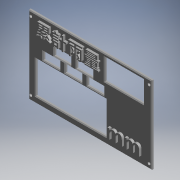
# Autodesk Inventor part: 雨量
Saved by Autodesk Inventor 2021 (Build 250183000, 183)
## iProperties
Part Number: 雨量
Material: 一般
Document SubType Name: 塑型
Designer: aura0
Appearance: 預設
Author: aura0
Autodesk Inventor part; units mm, degrees
ref_plane "YZ 平面" through (0, 0, 0) normal (1, 0, 0) x (0, 1, 0)
ref_plane "XZ 平面" through (0, 0, 0) normal (0, 1, 0) x (-1, 0, 0)
ref_plane "XY 平面" through (0, 0, 0) normal (0, 0, 1) x (1, 0, 0)
sketch "草圖1" plane through (0, 0, 0) normal (0, 0, 1) x (1, 0, 0)
  line L0 (-81, -51) -> (81, -51)
  line L1 (81, -51) -> (81, 51)
  line L2 (81, 51) -> (-81, 51)
  line L3 (-81, 51) -> (-81, -51)
  line L4 (-81, -51) -> (81, 51) construction
  line L5 (81, -51) -> (-81, 51) construction
  point P0 (0, 0)
  dimension "d0" = 162
  dimension "d1" = 102
  constraints: 12 end point, 2 midpoint, 2 parallel, 1 horizontal, 1 perpendicular
  measures "d0" distance of L2.end L1.end
  measures "d1" distance of L1.end L0.end
extrude "擠出1" add sketch "草圖1" along normal blind 3
sketch "草圖2" plane through (0, 0, 3) normal (0, 0, 1) x (1, 0, 0)
  line L0 (-72, -43) -> (21, -43)
  line L1 (21, -43) -> (21, 0)
  line L2 (21, 0) -> (-72, 0)
  line L3 (-72, 0) -> (-72, -43)
  line L4 (-62, 2.8) -> (-40, 2.8)
  line L5 (-40, 2.8) -> (-40, 13)
  line L6 (-40, 13) -> (-62, 13)
  line L7 (-62, 13) -> (-62, 2.8)
  line L8 (-33, 2.8) -> (-11, 2.8)
  line L9 (-11, 2.8) -> (-11, 13)
  line L10 (-11, 13) -> (-33, 13)
  line L11 (-33, 13) -> (-33, 2.8)
  line L12 (-4, 2.8) -> (18, 2.8)
  line L13 (18, 2.8) -> (18, 13)
  line L14 (18, 13) -> (-4, 13)
  line L15 (-4, 13) -> (-4, 2.8)
  line L16 (-47.5, 15) -> (-25.5, 15)
  line L17 (-25.5, 15) -> (-25.5, 25.2)
  line L18 (-25.5, 25.2) -> (-47.5, 25.2)
  line L19 (-47.5, 25.2) -> (-47.5, 15)
  line L20 (-18.5, 15) -> (3.5, 15)
  line L21 (3.5, 15) -> (3.5, 25.2)
  line L22 (3.5, 25.2) -> (-18.5, 25.2)
  line L23 (-18.5, 25.2) -> (-18.5, 15)
  line L24 (19, 19) -> (70, 19)
  line L25 (70, 19) -> (70, 47)
  line L26 (70, 47) -> (19, 47)
  line L27 (19, 47) -> (19, 19)
  line L28 (-81, -51) -> (81, -51) projected
  line L29 (-81, 51) -> (-81, -51) projected
  point P0 (0, 0)
  dimension "d4" = 8
  dimension "d5" = 9
  dimension "d6" = 43
  dimension "d7" = 93
  dimension "d8" = 53.8
  dimension "d9" = 19
  dimension "d10" = 22
  dimension "d11" = 10.2
  dimension "d12" = 0
  dimension "d13" = 0
  dimension "d14" = 22
  dimension "d15" = 7
  dimension "d16" = 7
  dimension "d17" = 22
  dimension "d18" = 10.2
  dimension "d19" = 10.2
  dimension "d20" = 66
  dimension "d21" = 33.5
  dimension "d22" = 22
  dimension "d23" = 10.2
  dimension "d24" = 0
  dimension "d25" = 7
  dimension "d26" = 22
  dimension "d27" = 10.2
  dimension "d28" = 70
  dimension "d29" = 100
  dimension "d30" = 51
  dimension "d31" = 28
  constraints: 56 end point, 14 parallel, 7 horizontal, 7 perpendicular
  measures "d4" distance between parallel lines of L28 L0
  measures "d5" distance between parallel lines of L29 L3
  measures "d6" distance of L0.end L1.end
  measures "d7" distance of L0.start L0.end
  measures "d8" distance between parallel lines of L28 L4
  measures "d9" distance between parallel lines of L29 L7
  measures "d10" distance of L4.start L4.end
  measures "d11" distance of L4.end L5.end
  measures "d12" distance between parallel lines of L4 L8
  measures "d13" distance between parallel lines of L4 L12
  measures "d14" distance of L8.start L8.end
  measures "d15" distance between parallel lines of L5 L11
  measures "d16" distance between parallel lines of L15 L9
  measures "d17" distance of L12.start L12.end
  measures "d18" distance of L8.end L9.end
  measures "d19" distance of L12.end L13.end
  measures "d20" distance between parallel lines of L28 L16
  measures "d21" distance between parallel lines of L29 L19
  measures "d22" distance of L16.start L16.end
  measures "d23" distance of L16.end L17.end
  measures "d24" distance between parallel lines of L16 L20
  measures "d25" distance between parallel lines of L23 L17
  measures "d26" distance of L20.start L20.end
  measures "d27" distance of L20.end L21.end
  measures "d28" distance between parallel lines of L28 L24
  measures "d29" distance between parallel lines of L27 L29
  measures "d30" distance of L24.start L24.end
  measures "d31" distance of L24.end L25.end
extrude "擠出2" cut sketch "草圖2" against normal blind 3
sketch "草圖3" plane through (0, 0, 3) normal (0, 0, 1) x (1, 0, 0)
  line L0 (-69.5952, 46.7883) -> (36.1559, 46.7883) construction
  line L1 (36.1559, 46.7883) -> (36.1559, 23.2347) construction
  line L2 (36.1559, 23.2347) -> (-69.5952, 23.2347) construction
  line L3 (-69.5952, 23.2347) -> (-69.5952, 46.7883) construction
  line L4 (23.9815, -27.7989) -> (32.0649, -27.7989) construction
  line L5 (32.0649, -27.7989) -> (32.0649, -30.4991) construction
  line L6 (32.0649, -30.4991) -> (23.9815, -30.4991) construction
  line L7 (23.9815, -30.4991) -> (23.9815, -27.7989) construction
  line L8 (-50.1617, 32.9995) -> (-51.6312, 31.9832)
  spline S0 degree 2 poles (-51.6312, 31.9832) (-52.2355, 32.7935) (-52.7574, 33.3016) knots 0 0 0 1 1 1
  spline S1 degree 2 poles (-52.7574, 33.3016) (-55.1609, 33.0132) (-57.9214, 32.8759) knots 0 0 0 1 1 1
  line L9 (-57.9214, 32.8759) -> (-57.9214, 30.0467)
  spline S2 degree 2 poles (-57.9214, 30.0467) (-57.9214, 29.2776) (-58.8553, 28.1377) (-60.6682, 28.1377) knots 0 0 0 1 2 2 2
  spline S3 degree 2 poles (-60.6682, 28.1377) (-61.1626, 28.1377) (-61.6158, 28.1789) knots 0 0 0 1 1 1
  line L10 (-61.6158, 28.1789) -> (-62.2338, 29.7858)
  spline S4 degree 2 poles (-62.2338, 29.7858) (-60.8467, 29.7583) (-59.7892, 29.8407) (-59.7892, 30.2939) knots 0 0 0 1 2 2 2
  line L11 (-59.7892, 30.2939) -> (-59.7892, 32.7248)
  spline S5 degree 2 poles (-59.7892, 32.7248) (-63.4012, 32.4913) (-66.7797, 32.4913) knots 0 0 0 1 1 1
  line L12 (-66.7797, 32.4913) -> (-67.1231, 34.0021)
  spline S6 degree 2 poles (-67.1231, 34.0021) (-64.1566, 34.263) (-59.8716, 36.0759) knots 0 0 0 1 1 1
  spline S7 degree 2 poles (-59.8716, 36.0759) (-64.5411, 35.6639) (-65.5574, 35.6227) knots 0 0 0 1 1 1
  line L13 (-65.5574, 35.6227) -> (-65.7909, 37.1059)
  spline S8 degree 2 poles (-65.7909, 37.1059) (-63.6484, 37.5729) (-61.5197, 39.0424) knots 0 0 0 1 1 1
  line L14 (-61.5197, 39.0424) -> (-66.3815, 39.0424)
  line L15 (-66.3815, 39.0424) -> (-66.3815, 46.239)
  line L16 (-66.3815, 46.239) -> (-51.4527, 46.239)
  line L17 (-51.4527, 46.239) -> (-51.4527, 39.0424)
  line L18 (-51.4527, 39.0424) -> (-58.8965, 39.0424)
  spline S9 degree 2 poles (-58.8965, 39.0424) (-60.3385, 37.9025) (-61.8081, 37.2158) knots 0 0 0 1 1 1
  spline S10 degree 2 poles (-61.8081, 37.2158) (-60.833, 37.2433) (-58.9102, 37.3806) (-56.4793, 37.6415) (-55.5729, 38.1222) (-54.8724, 38.548) knots 0 0 0 1 2 3 4 4 4
  line L19 (-54.8724, 38.548) -> (-53.2656, 37.669)
  spline S11 degree 2 poles (-53.2656, 37.669) (-57.5368, 35.3343) (-62.0003, 34.0021) knots 0 0 0 1 1 1
  spline S12 degree 2 poles (-62.0003, 34.0021) (-58.0587, 34.1257) (-54.1308, 34.6064) knots 0 0 0 1 1 1
  spline S13 degree 2 poles (-54.1308, 34.6064) (-54.2956, 34.7986) (-55.0235, 35.4167) knots 0 0 0 1 1 1
  line L20 (-55.0235, 35.4167) -> (-53.5265, 36.378)
  spline S14 degree 2 poles (-53.5265, 36.378) (-51.5488, 34.7574) (-50.1617, 32.9995) knots 0 0 0 1 1 1
  line L21 (-49.5849, 29.7583) -> (-50.7111, 28.3712)
  spline S15 degree 2 poles (-50.7111, 28.3712) (-53.293, 29.9231) (-56.6167, 31.0493) knots 0 0 0 1 1 1
  line L22 (-56.6167, 31.0493) -> (-55.2982, 32.3815)
  spline S16 degree 2 poles (-55.2982, 32.3815) (-51.9883, 31.2553) (-49.5849, 29.7583) knots 0 0 0 1 1 1
  spline S17 degree 2 poles (-61.0939, 31.2003) (-63.4699, 29.6347) (-67.1643, 28.4536) knots 0 0 0 1 1 1
  line L23 (-67.1643, 28.4536) -> (-68.2767, 29.978)
  spline S18 degree 2 poles (-68.2767, 29.978) (-64.9531, 30.8845) (-62.7145, 32.2441) knots 0 0 0 1 1 1
  line L24 (-62.7145, 32.2441) -> (-61.0939, 31.2003)
  line L25 (-53.3342, 43.3823) -> (-53.3342, 44.6596)
  line L26 (-53.3342, 44.6596) -> (-58.0038, 44.6596)
  line L27 (-58.0038, 44.6596) -> (-58.0038, 43.3823)
  line L28 (-58.0038, 43.3823) -> (-53.3342, 43.3823)
  line L29 (-53.3342, 40.663) -> (-53.3342, 41.9265)
  line L30 (-53.3342, 41.9265) -> (-58.0038, 41.9265)
  line L31 (-58.0038, 41.9265) -> (-58.0038, 40.663)
  line L32 (-58.0038, 40.663) -> (-53.3342, 40.663)
  line L33 (-59.8853, 43.3823) -> (-59.8853, 44.6596)
  line L34 (-59.8853, 44.6596) -> (-64.4587, 44.6596)
  line L35 (-64.4587, 44.6596) -> (-64.4587, 43.3823)
  line L36 (-64.4587, 43.3823) -> (-59.8853, 43.3823)
  line L37 (-59.8853, 40.663) -> (-59.8853, 41.9265)
  line L38 (-59.8853, 41.9265) -> (-64.4587, 41.9265)
  line L39 (-64.4587, 41.9265) -> (-64.4587, 40.663)
  line L40 (-64.4587, 40.663) -> (-59.8853, 40.663)
  line L41 (-28.5583, 38.9463) -> (-32.4175, 38.9463)
  line L42 (-32.4175, 38.9463) -> (-32.4175, 28.1789)
  line L43 (-32.4175, 28.1789) -> (-34.3403, 28.1789)
  line L44 (-34.3403, 28.1789) -> (-34.3403, 38.9463)
  line L45 (-34.3403, 38.9463) -> (-38.1033, 38.9463)
  line L46 (-38.1033, 38.9463) -> (-38.1033, 40.8003)
  line L47 (-38.1033, 40.8003) -> (-34.3403, 40.8003)
  line L48 (-34.3403, 40.8003) -> (-34.3403, 46.6235)
  line L49 (-34.3403, 46.6235) -> (-32.4175, 46.6235)
  line L50 (-32.4175, 46.6235) -> (-32.4175, 40.8003)
  line L51 (-32.4175, 40.8003) -> (-28.5583, 40.8003)
  line L52 (-28.5583, 40.8003) -> (-28.5583, 38.9463)
  line L53 (-39.1746, 28.4536) -> (-41.0149, 28.4536)
  line L54 (-41.0149, 28.4536) -> (-41.0149, 29.5111)
  line L55 (-41.0149, 29.5111) -> (-44.2973, 29.5111)
  line L56 (-44.2973, 29.5111) -> (-44.2973, 28.1789)
  line L57 (-44.2973, 28.1789) -> (-46.1651, 28.1789)
  line L58 (-46.1651, 28.1789) -> (-46.1651, 35.4579)
  line L59 (-46.1651, 35.4579) -> (-39.1746, 35.4579)
  line L60 (-39.1746, 35.4579) -> (-39.1746, 28.4536)
  line L61 (-38.227, 43.039) -> (-47.0304, 43.039)
  line L62 (-47.0304, 43.039) -> (-47.0304, 44.7145)
  line L63 (-47.0304, 44.7145) -> (-43.542, 44.7145)
  spline S19 degree 2 poles (-43.542, 44.7145) (-43.8853, 45.6072) (-44.3248, 46.4312) knots 0 0 0 1 1 1
  line L64 (-44.3248, 46.4312) -> (-42.3471, 46.7883)
  spline S20 degree 2 poles (-42.3471, 46.7883) (-41.8664, 45.9368) (-41.427, 44.7145) knots 0 0 0 1 1 1
  line L65 (-41.427, 44.7145) -> (-38.227, 44.7145)
  line L66 (-38.227, 44.7145) -> (-38.227, 43.039)
  line L67 (-39.2158, 39.8939) -> (-46.2613, 39.8939)
  line L68 (-46.2613, 39.8939) -> (-46.2613, 41.5832)
  line L69 (-46.2613, 41.5832) -> (-39.2158, 41.5832)
  line L70 (-39.2158, 41.5832) -> (-39.2158, 39.8939)
  line L71 (-39.2158, 36.845) -> (-46.2613, 36.845)
  line L72 (-46.2613, 36.845) -> (-46.2613, 38.5205)
  line L73 (-46.2613, 38.5205) -> (-39.2158, 38.5205)
  line L74 (-39.2158, 38.5205) -> (-39.2158, 36.845)
  line L75 (-41.0149, 31.2003) -> (-41.0149, 33.7137)
  line L76 (-41.0149, 33.7137) -> (-44.2973, 33.7137)
  line L77 (-44.2973, 33.7137) -> (-44.2973, 31.2003)
  line L78 (-44.2973, 31.2003) -> (-41.0149, 31.2003)
  line L79 (-7.4905, 44.2888) -> (-15.6896, 44.2888)
  line L80 (-15.6896, 44.2888) -> (-15.6896, 42.2424)
  line L81 (-15.6896, 42.2424) -> (-8.4244, 42.2424)
  line L82 (-8.4244, 42.2424) -> (-8.4244, 30.5961)
  spline S21 degree 2 poles (-8.4244, 30.5961) (-8.4244, 29.1677) (-9.7428, 28.1926) (-11.1162, 28.1926) knots 0 0 0 1 2 2 2
  spline S22 degree 2 poles (-11.1162, 28.1926) (-11.542, 28.1926) (-12.16, 28.2476) knots 0 0 0 1 1 1
  line L83 (-12.16, 28.2476) -> (-12.778, 30.0879)
  spline S23 degree 2 poles (-12.778, 30.0879) (-11.954, 30.033) (-11.5008, 30.033) knots 0 0 0 1 1 1
  spline S24 degree 2 poles (-11.5008, 30.033) (-10.663, 30.033) (-10.251, 30.3076) (-10.251, 30.651) knots 0 0 0 1 2 2 2
  line L84 (-10.251, 30.651) -> (-10.251, 40.4433)
  line L85 (-10.251, 40.4433) -> (-15.6896, 40.4433)
  line L86 (-15.6896, 40.4433) -> (-15.6896, 28.6321)
  line L87 (-15.6896, 28.6321) -> (-17.5437, 28.6321)
  line L88 (-17.5437, 28.6321) -> (-17.5437, 40.4433)
  line L89 (-17.5437, 40.4433) -> (-22.9411, 40.4433)
  line L90 (-22.9411, 40.4433) -> (-22.9411, 28.1377)
  line L91 (-22.9411, 28.1377) -> (-24.8227, 28.1377)
  line L92 (-24.8227, 28.1377) -> (-24.8227, 42.2424)
  line L93 (-24.8227, 42.2424) -> (-17.5437, 42.2424)
  line L94 (-17.5437, 42.2424) -> (-17.5437, 44.2888)
  line L95 (-17.5437, 44.2888) -> (-25.8802, 44.2888)
  line L96 (-25.8802, 44.2888) -> (-25.8802, 46.1291)
  line L97 (-25.8802, 46.1291) -> (-7.4905, 46.1291)
  line L98 (-7.4905, 46.1291) -> (-7.4905, 44.2888)
  spline S25 degree 2 poles (-18.2441, 33.8235) (-19.439, 32.1205) (-21.1969, 30.4862) knots 0 0 0 1 1 1
  line L99 (-21.1969, 30.4862) -> (-22.5154, 31.8596)
  spline S26 degree 2 poles (-22.5154, 31.8596) (-20.7437, 33.5076) (-19.6999, 35.0046) knots 0 0 0 1 1 1
  line L100 (-19.6999, 35.0046) -> (-18.2441, 33.8235)
  line L101 (-10.6905, 31.7497) -> (-12.2149, 30.6373)
  spline S27 degree 2 poles (-12.2149, 30.6373) (-13.039, 31.9832) (-14.9068, 33.9197) knots 0 0 0 1 1 1
  line L102 (-14.9068, 33.9197) -> (-13.4235, 35.0458)
  spline S28 degree 2 poles (-13.4235, 35.0458) (-11.7892, 33.3428) (-10.6905, 31.7497) knots 0 0 0 1 1 1
  spline S29 degree 2 poles (-10.9514, 38.9463) (-12.1325, 36.9549) (-13.3686, 35.5815) knots 0 0 0 1 1 1
  line L103 (-13.3686, 35.5815) -> (-14.8793, 36.6664)
  spline S30 degree 2 poles (-14.8793, 36.6664) (-13.7669, 37.8613) (-12.5583, 39.8527) knots 0 0 0 1 1 1
  line L104 (-12.5583, 39.8527) -> (-10.9514, 38.9463)
  line L105 (-18.4501, 36.6802) -> (-20.0158, 35.6639)
  spline S31 degree 2 poles (-20.0158, 35.6639) (-20.9497, 37.3394) (-22.3506, 38.9051) knots 0 0 0 1 1 1
  line L106 (-22.3506, 38.9051) -> (-20.7574, 39.8939)
  spline S32 degree 2 poles (-20.7574, 39.8939) (-19.233, 38.1909) (-18.4501, 36.6802) knots 0 0 0 1 1 1
  line L107 (13.7421, 28.4673) -> (-4.6613, 28.4673)
  line L108 (-4.6613, 28.4673) -> (-4.6613, 29.7995)
  line L109 (-4.6613, 29.7995) -> (3.6203, 29.7995)
  line L110 (3.6203, 29.7995) -> (3.6203, 30.7609)
  line L111 (3.6203, 30.7609) -> (-3.4115, 30.7609)
  line L112 (-3.4115, 30.7609) -> (-3.4115, 31.942)
  line L113 (-3.4115, 31.942) -> (3.6203, 31.942)
  line L114 (3.6203, 31.942) -> (3.6203, 32.8484)
  line L115 (3.6203, 32.8484) -> (-3.0132, 32.8484)
  line L116 (-3.0132, 32.8484) -> (-3.0132, 38.0124)
  line L117 (-3.0132, 38.0124) -> (12.0391, 38.0124)
  line L118 (12.0391, 38.0124) -> (12.0391, 32.8484)
  line L119 (12.0391, 32.8484) -> (5.4057, 32.8484)
  line L120 (5.4057, 32.8484) -> (5.4057, 31.942)
  line L121 (5.4057, 31.942) -> (12.616, 31.942)
  line L122 (12.616, 31.942) -> (12.616, 30.7334)
  line L123 (12.616, 30.7334) -> (5.4057, 30.7334)
  line L124 (5.4057, 30.7334) -> (5.4057, 29.7995)
  line L125 (5.4057, 29.7995) -> (13.7421, 29.7995)
  line L126 (13.7421, 29.7995) -> (13.7421, 28.4673)
  line L127 (12.0254, 41.1849) -> (-3.0407, 41.1849)
  line L128 (-3.0407, 41.1849) -> (-3.0407, 46.39)
  line L129 (-3.0407, 46.39) -> (12.0254, 46.39)
  line L130 (12.0254, 46.39) -> (12.0254, 41.1849)
  line L131 (13.5636, 38.8776) -> (-4.5102, 38.8776)
  line L132 (-4.5102, 38.8776) -> (-4.5102, 40.3334)
  line L133 (-4.5102, 40.3334) -> (13.5636, 40.3334)
  line L134 (13.5636, 40.3334) -> (13.5636, 38.8776)
  line L135 (10.1988, 42.3935) -> (10.1988, 43.2587)
  line L136 (10.1988, 43.2587) -> (-1.2553, 43.2587)
  line L137 (-1.2553, 43.2587) -> (-1.2553, 42.3935)
  line L138 (-1.2553, 42.3935) -> (10.1988, 42.3935)
  line L139 (10.1988, 44.3986) -> (10.1988, 45.1815)
  line L140 (10.1988, 45.1815) -> (-1.2553, 45.1815)
  line L141 (-1.2553, 45.1815) -> (-1.2553, 44.3986)
  line L142 (-1.2553, 44.3986) -> (10.1988, 44.3986)
  line L143 (3.6203, 35.9797) -> (3.6203, 36.845)
  line L144 (3.6203, 36.845) -> (-1.2415, 36.845)
  line L145 (-1.2415, 36.845) -> (-1.2415, 35.9797)
  line L146 (-1.2415, 35.9797) -> (3.6203, 35.9797)
  line L147 (3.6203, 34.0158) -> (3.6203, 34.881)
  line L148 (3.6203, 34.881) -> (-1.2141, 34.881)
  line L149 (-1.2141, 34.881) -> (-1.2415, 34.0158)
  line L150 (-1.2415, 34.0158) -> (3.6203, 34.0158)
  line L151 (10.2263, 34.0158) -> (10.2263, 34.881)
  line L152 (10.2263, 34.881) -> (5.4057, 34.881)
  line L153 (5.4057, 34.881) -> (5.4057, 34.0158)
  line L154 (5.4057, 34.0158) -> (10.2263, 34.0158)
  line L155 (10.2263, 35.9797) -> (10.2263, 36.845)
  line L156 (10.2263, 36.845) -> (5.4057, 36.845)
  line L157 (5.4057, 36.845) -> (5.4057, 35.9797)
  line L158 (5.4057, 35.9797) -> (10.2263, 35.9797)
  line L159 (44.9171, -40.9474) -> (42.1823, -40.9474)
  line L160 (42.1823, -40.9474) -> (42.1823, -33.5775)
  spline S33 degree 2 poles (42.1823, -33.5775) (42.1823, -31.677) (40.9617, -29.9775) (39.6021, -29.9775) knots 0 0 0 1 2 2 2
  spline S34 degree 2 poles (39.6021, -29.9775) (38.4433, -29.9775) (36.7746, -32.1251) (36.7746, -33.6702) knots 0 0 0 1 2 2 2
  line L161 (36.7746, -33.6702) -> (36.7746, -40.9474)
  line L162 (36.7746, -40.9474) -> (34.0553, -40.9474)
  line L163 (34.0553, -40.9474) -> (34.0553, -33.3921)
  spline S35 degree 2 poles (34.0553, -33.3921) (34.0553, -29.9775) (31.4441, -29.9775) knots 0 0 0 1 1 1
  spline S36 degree 2 poles (31.4441, -29.9775) (30.239, -29.9775) (28.6476, -32.0478) (28.6476, -33.6856) knots 0 0 0 1 2 2 2
  line L164 (28.6476, -33.6856) -> (28.6476, -40.9474)
  line L165 (28.6476, -40.9474) -> (25.9128, -40.9474)
  line L166 (25.9128, -40.9474) -> (25.9128, -28.0925)
  line L167 (25.9128, -28.0925) -> (28.6476, -28.0925)
  line L168 (28.6476, -28.0925) -> (28.6476, -30.1165)
  line L169 (28.6476, -30.1165) -> (28.6939, -30.1165)
  spline S37 degree 2 poles (28.6939, -30.1165) (30.0845, -27.7989) (32.742, -27.7989) knots 0 0 0 1 1 1
  spline S38 degree 2 poles (32.742, -27.7989) (35.4458, -27.7989) (36.4038, -30.3637) knots 0 0 0 1 1 1
  spline S39 degree 2 poles (36.4038, -30.3637) (37.8407, -27.7989) (40.6991, -27.7989) knots 0 0 0 1 1 1
  spline S40 degree 2 poles (40.6991, -27.7989) (44.9171, -27.7989) (44.9171, -33.0058) knots 0 0 0 1 1 1
  line L170 (44.9171, -33.0058) -> (44.9171, -40.9474)
  line L171 (67.5368, -40.9474) -> (64.8021, -40.9474)
  line L172 (64.8021, -40.9474) -> (64.8021, -33.5775)
  spline S41 degree 2 poles (64.8021, -33.5775) (64.8021, -31.677) (63.5815, -29.9775) (62.2218, -29.9775) knots 0 0 0 1 2 2 2
  spline S42 degree 2 poles (62.2218, -29.9775) (61.063, -29.9775) (59.3943, -32.1251) (59.3943, -33.6702) knots 0 0 0 1 2 2 2
  line L173 (59.3943, -33.6702) -> (59.3943, -40.9474)
  line L174 (59.3943, -40.9474) -> (56.675, -40.9474)
  line L175 (56.675, -40.9474) -> (56.675, -33.3921)
  spline S43 degree 2 poles (56.675, -33.3921) (56.675, -29.9775) (54.0639, -29.9775) knots 0 0 0 1 1 1
  spline S44 degree 2 poles (54.0639, -29.9775) (52.8587, -29.9775) (51.2673, -32.0478) (51.2673, -33.6856) knots 0 0 0 1 2 2 2
  line L176 (51.2673, -33.6856) -> (51.2673, -40.9474)
  line L177 (51.2673, -40.9474) -> (48.5325, -40.9474)
  line L178 (48.5325, -40.9474) -> (48.5325, -28.0925)
  line L179 (48.5325, -28.0925) -> (51.2673, -28.0925)
  line L180 (51.2673, -28.0925) -> (51.2673, -30.1165)
  line L181 (51.2673, -30.1165) -> (51.3137, -30.1165)
  spline S45 degree 2 poles (51.3137, -30.1165) (52.7042, -27.7989) (55.3617, -27.7989) knots 0 0 0 1 1 1
  spline S46 degree 2 poles (55.3617, -27.7989) (58.0656, -27.7989) (59.0235, -30.3637) knots 0 0 0 1 1 1
  spline S47 degree 2 poles (59.0235, -30.3637) (60.4604, -27.7989) (63.3188, -27.7989) knots 0 0 0 1 1 1
  spline S48 degree 2 poles (63.3188, -27.7989) (67.5368, -27.7989) (67.5368, -33.0058) knots 0 0 0 1 1 1
  line L182 (67.5368, -33.0058) -> (67.5368, -40.9474)
  point P0 (0, 0)
  constraints: 4 other
extrude "擠出3" add sketch "草圖3" along normal blind 3
sketch "草圖4" plane through (0, 0, 3) normal (0, 0, 1) x (1, 0, 0)
  circle A0 centre (-77.9, -45) radius 1.8
  circle A1 centre (77.7, -45) radius 1.8
  circle A2 centre (77.7, 45) radius 1.8
  circle A3 centre (-77.9, 45) radius 1.8
  line L0 (-81, -51) -> (81, -51) projected
  line L1 (-81, 51) -> (-81, -51) projected
  point P0 (0, 0)
  dimension "d36" = 6
  dimension "d37" = 6
  dimension "d38" = 96
  dimension "d39" = 96
  dimension "d40" = 158.7
  dimension "d41" = 158.7
  dimension "d42" = 3.1
  dimension "d43" = 3.1
  dimension "d44" = 3.6
  dimension "d45" = 3.6
  dimension "d46" = 3.6
  dimension "d47" = 3.6
  constraints: 4 centre point
  measures "d36" distance from line of L0 A0.centre
  measures "d37" distance from line of L0 A1.centre
  measures "d38" distance from line of L0 A3.centre
  measures "d39" distance from line of L0 A2.centre
  measures "d40" distance from line of L1 A1.centre
  measures "d41" distance from line of L1 A2.centre
  measures "d42" distance from line of L1 A3.centre
  measures "d43" distance from line of L1 A0.centre
  measures "d44" diameter of A3
  measures "d45" diameter of A0
  measures "d46" diameter of A1
  measures "d47" diameter of A2
extrude "擠出4" cut sketch "草圖4" against normal blind 3
chamfer "倒角1" distance 1 angle 45 32 edges at (-36.5, 15, 3) (-47.5, 20.1, 3) (-36.5, 25.2, 3) (-25.5, 20.1, 3) (-18.5, 20.1, 3) (-7.5, 25.2, 3) (3.5, 20.1, 3) (-7.5, 15, 3) (7, 13, 3) (18, 7.9, 3) (7, 2.8, 3) (-4, 7.9, 3) (-11, 7.9, 3) (-22, 13, 3) (-22, 2.8, 3) (-33, 7.9, 3) (-40, 7.9, 3) (-51, 13, 3) (-62, 7.9, 3) (-51, 2.8, 3) (-25.5, 0, 3) (-72, -21.5, 3) (-25.5, -43, 3) (21, -21.5, 3) (-81, 0, 3) (0, 51, 3) (81, 0, 3) (0, -51, 3) (44.5, 19, 3) (19, 33, 3) (44.5, 47, 3) (70, 33, 3)
equation "\"d14\" = d10"
equation "\"d17\" = d10"
equation "\"d18\" = d11"
equation "\"d19\" = d11"
equation "\"d22\" = d10"
equation "\"d23\" = d11"
equation "\"d25\" = d15"
equation "\"d26\" = d10"
equation "\"d27\" = d11"
